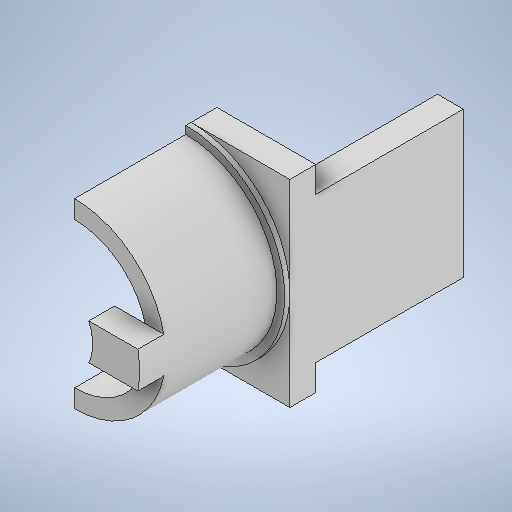
# Autodesk Inventor part: j4 motor mount cover
Saved by Autodesk Inventor 2025 (Build 290162000, 162)
## iProperties
Created: 2025-08-04
Part Number: j4 motor mount cover
Material: 一般
Document SubType Name: Modeling
Designer: gavin
Density: 1 g/cm^3
Appearance: 預設
Author: gavin
## iProperties of the stored document j4 motor mount cover_3D 列印.ipt
Created: 2025-08-05
Part Number: j4 motor mount cover_3D 列印
Material: 一般
Document SubType Name: Modeling
Designer: gavin
Density: 1 g/cm^3
Appearance: 預設
Author: gavin
Autodesk Inventor part; units mm, degrees
ref_plane "YZ Plane" through (0, 0, 0) normal (1, 0, 0) x (0, 1, 0)
ref_plane "XZ Plane" through (0, 0, 0) normal (0, 1, 0) x (-1, 0, 0)
ref_plane "XY Plane" through (0, 0, 0) normal (0, 0, 1) x (1, 0, 0)
ref_plane "工作平面1" through (0, 0, -40) normal (0, 0, -1) x (-1, 0, 0)
sketch "草圖1" plane through (0, 0, -40) normal (0, 0, -1) x (-1, 0, 0)
  line L0 (-15.075, 14.075) -> (-15.075, 19.075) projected
  line L1 (-19.075, 19.075) -> (-15.075, 19.075) projected
  line L2 (-19.075, 14.075) -> (-19.075, 19.075) projected
  line L3 (-15.075, 14.075) -> (-19.075, 14.075) projected
  line L4 (-15.075, -19.075) -> (-15.075, -14.075) projected
  line L5 (-19.075, -14.075) -> (-15.075, -14.075) projected
  line L6 (-19.075, -19.075) -> (-19.075, -14.075) projected
  line L7 (-15.075, -19.075) -> (-19.075, -19.075) projected
  line L8 (-19.075, 14.075) -> (-19.075, -14.075)
  line L9 (-15.075, -14.075) -> (-15.075, 14.075)
  point P0 (0, 0)
  constraints: 4 end point, 2 point on line, 1 perpendicular, 1 vertical
extrude "擠出1" add sketch "草圖1" along normal blind 5
sketch "草圖2" plane through (0, 0, -40) normal (0, 0, 1) x (1, 0, 0)
  line L0 (15.075, -19.075) -> (15.075, 19.075) projected
  line L1 (19.075, -19.075) -> (15.075, -19.075) projected
  line L2 (19.075, 19.075) -> (19.075, -19.075) projected
  line L3 (15.075, 19.075) -> (19.075, 19.075) projected
  line L4 (0, 14.075) -> (19.075, 14.075) projected
  line L5 (19.075, -14.075) -> (0, -14.075) projected
  point P0 (0, 0)
  point P1 (15.075, -14.075)
  point P2 (15.075, 14.075)
ref_plane "工作平面2" through (0, -19.075, 0) normal (0, 0, 1) x (1, 0, 0)
extrude "擠出2" add sketch "草圖2" along normal up to surface (40 mm away) contours L0 L4 L2 L5
sketch "草圖3" plane through (15.075, -14.075, 0) normal (0, 0, 1) x (1, 0, 0)
  line L0 (-15.075, 33.15) -> (-15.075, 28.15) projected
  line L1 (-15.075, 28.15) -> (4, 28.15) projected
  line L2 (4, 28.15) -> (4, 33.15) projected
  line L3 (4, 33.15) -> (-15.075, 33.15) projected
  line L4 (4, 0) -> (0, 0) projected
  line L5 (4, 28.15) -> (4, 0) projected
  line L6 (0, 28.15) -> (4, 28.15) projected
  line L7 (0, 0) -> (0, 28.15) projected
  line L8 (-15.075, 0) -> (-15.075, -5) projected
  line L9 (-15.075, -5) -> (4, -5) projected
  line L10 (4, -5) -> (4, 0) projected
  line L11 (4, 0) -> (-15.075, 0) projected
  point P0 (-15.075, 14.075)
  point P1 (0, 28.15)
  point P2 (4, 28.15)
ref_plane "工作平面3" through (-19.075, 0, 5) normal (0, 0, 1) x (1, 0, 0)
extrude "擠出3" add sketch "草圖3" along normal up to surface (5 mm away)
sketch "草圖4" plane through (0, -19.075, 5) normal (0, 0, 1) x (1, 0, 0)
  arc A0 (0, 38.15) -> (0, 0) centre (0, 19.075) ccw projected
  circle A1 centre (0, 19.075) radius 19.075
  arc A2 (0, 36.65) -> (0, 1.5) centre (0, 19.075) ccw projected
  circle A3 centre (0, 19.075) radius 17.575
  line L0 (0, 38.15) -> (0, 33.15) projected
  line L1 (0, 38.15) -> (0, 0)
  point P0 (0, 1.5)
  point P1 (0, 38.15)
  point P2 (0, 1.5)
  point P3 (0, 38.15)
  constraints: 2 coincident, 2 end point, 1 collinear, 6 other
extrude "擠出4" add sketch "草圖4" along normal blind 1 contours A1 L1 A3 L0
sketch "草圖5" plane through (15.075, -14.075, 0) normal (0, 0, -1) x (-1, 0, 0)
  arc A0 (15.075, 0) -> (15.075, 28.15) centre (15.075, 14.075) ccw projected
  circle A1 centre (15.075, 14.075) radius 14.075
  line L0 (15.075, 28.15) -> (-4, 28.15) projected
  line L1 (0, -5) -> (0, 33.15) projected
  line L2 (-4, 0) -> (15.075, 0) projected
  point P0 (0, 0)
  point P1 (15.075, 28.15)
  point P2 (0, 28.15)
  constraints: 1 coincident, 3 other
extrude "擠出5" add sketch "草圖5" against normal up to surface (5 mm away) contours L2 L1 L0 A1
sketch "草圖6" plane through (0, 0, 5) normal (0, 0, 1) x (1, 0, 0)
  arc A0 (0, -17.575) -> (0, 17.575) centre (0, 0) ccw projected
  line L0 (0, 14.075) -> (0, 17.575) projected
  arc A1 (0, -14.075) -> (0, 14.075) centre (0, 0) ccw projected
  line L1 (0, -17.575) -> (0, -14.075) projected
ref_plane "工作平面4" through (-14.075, -17.575, 27.5) normal (0, 0, -1) x (0, 1, 0)
extrude "擠出6" add sketch "草圖6" along normal up to surface (22.5 mm away)
sketch "草圖7" plane through (0, 0, 27.5) normal (0, 0, 1) x (1, 0, 0)
  line L0 (17.223, -3.5) -> (7.746, -3.5) projected
  arc A0 (7.746, 3.5) -> (7.746, -3.5) centre (0, 0) ccw projected
  line L1 (7.746, 3.5) -> (17.223, 3.5) projected
  arc A1 (17.223, 3.5) -> (17.223, -3.5) centre (0, 0) ccw projected
  circle A2 centre (7.7782, 7.7782) radius 1.6 projected
  circle A3 centre (-7.7782, 7.7782) radius 1.6 projected
  circle A4 centre (7.7782, -7.7782) radius 1.6 projected
  circle A5 centre (-7.7782, -7.7782) radius 1.6 projected
  arc A6 (0, -17.575) -> (0, 17.575) centre (0, 0) ccw projected
  circle A7 centre (0, 0) radius 8.5
  point P0 (7.746, -3.5)
  point P1 (7.746, 3.5)
  constraints: 1 centre point, 1 coincident
ref_plane "工作平面5" through (-17.575, -17.575, 32.5) normal (0, 0, 1) x (1, 0, 0)
extrude "擠出7" add sketch "草圖7" along normal up to surface (5 mm away) contours L0 A7 L1 A6
sketch "草圖8" plane through (15.075, -19.075, -45) normal (-1, 0, 0) x (0, 0, 1)
  line L0 (45, 5) -> (45, 33.15) projected
  line L1 (5, 33.15) -> (45, 33.15) projected
  line L2 (5, 33.15) -> (5, 38.15) projected
  line L3 (5, 38.15) -> (0, 38.15) projected
  line L4 (0, 0) -> (0, 38.15) projected
  line L5 (5, 0) -> (0, 0) projected
  line L6 (5, 0) -> (5, 5) projected
  line L7 (5, 5) -> (45, 5) projected
  point P0 (45, 19.075)
extrude "擠出8" add sketch "草圖8" along normal blind 1
sketch "草圖9" plane through (0, 0, -45) normal (0, 0, -1) x (-1, 0, 0)
  line L0 (-19.075, 19.075) -> (-14.075, 19.075) projected
  line L1 (-19.075, 19.075) -> (-19.075, -19.075) projected
  line L2 (-19.075, -19.075) -> (-14.075, -19.075) projected
  line L3 (-14.075, 19.075) -> (-14.075, -19.075) projected
  point P0 (0, 0)
extrude "擠出9" cut sketch "草圖9" against normal blind 16.5
